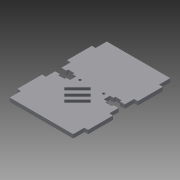
# Autodesk Inventor part: Motor_Mount_Front
Saved by Autodesk Inventor 2014 SP1 (Build 180222100, 222)
## iProperties
Created: 2014-03-20
Part Number: Motor_Mount_Front
Material: Generic
Document SubType Name: Modeling
Designer: ehagerup
Density: 1 g/cm^3
Appearance: Default
Author: ehagerup
Autodesk Inventor part; units mm, degrees
ref_plane "YZ Plane" through (0, 0, 0) normal (1, 0, 0) x (0, 1, 0)
ref_plane "XZ Plane" through (0, 0, 0) normal (0, 1, 0) x (-1, 0, 0)
ref_plane "XY Plane" through (0, 0, 0) normal (0, 0, 1) x (1, 0, 0)
sketch "Sketch1" plane through (0, 0, 0) normal (0, 0, 1) x (1, 0, 0)
  line L0 (0, 69) -> (3, 69)
  line L1 (3, 69) -> (3, 78)
  line L2 (3, 0) -> (3, 9)
  line L3 (3, 9) -> (0, 9)
  line L4 (0, 49) -> (3, 49)
  line L5 (3, 29) -> (0, 29)
  line L6 (15, 41.5) -> (15, 36.5)
  line L7 (12, 41.5) -> (12, 43)
  line L8 (12, 43) -> (7, 43)
  line L9 (7, 43) -> (7, 41.5)
  line L10 (12, 36.5) -> (12, 35)
  line L11 (12, 35) -> (7, 35)
  line L12 (7, 35) -> (7, 36.5)
  line L13 (0, 69) -> (0, 49)
  line L14 (0, 29) -> (0, 9)
  line L15 (3, 49) -> (3, 41.5)
  line L16 (3, 36.5) -> (3, 29)
  line L17 (15, 36.5) -> (12, 36.5)
  line L18 (7, 36.5) -> (3, 36.5)
  line L19 (3, 41.5) -> (7, 41.5)
  line L20 (12, 41.5) -> (15, 41.5)
  line L21 (57, 69) -> (54, 69)
  line L22 (54, 69) -> (54, 78)
  line L23 (54, 0) -> (54, 9)
  line L24 (54, 9) -> (57, 9)
  line L25 (57, 49) -> (54, 49)
  line L26 (54, 29) -> (57, 29)
  line L27 (42, 41.5) -> (42, 36.5)
  line L28 (45, 41.5) -> (45, 43)
  line L29 (45, 43) -> (50, 43)
  line L30 (50, 43) -> (50, 41.5)
  line L31 (45, 36.5) -> (45, 35)
  line L32 (45, 35) -> (50, 35)
  line L33 (50, 35) -> (50, 36.5)
  line L34 (57, 69) -> (57, 49)
  line L35 (57, 29) -> (57, 9)
  line L36 (54, 49) -> (54, 41.5)
  line L37 (54, 36.5) -> (54, 29)
  line L38 (42, 36.5) -> (45, 36.5)
  line L39 (50, 36.5) -> (54, 36.5)
  line L40 (54, 41.5) -> (50, 41.5)
  line L41 (45, 41.5) -> (42, 41.5)
  line L42 (3, 0) -> (54, 0)
  line L43 (54, 78) -> (3, 78)
  line L44 (24.2574, 22.636) -> (34.864, 33.2426)
  line L45 (34.864, 33.2426) -> (32.7426, 35.364)
  line L46 (32.7426, 35.364) -> (22.136, 24.7574)
  line L47 (22.136, 24.7574) -> (24.2574, 22.636)
  line L48 (20.0147, 26.8787) -> (30.6213, 37.4853)
  line L49 (30.6213, 37.4853) -> (28.5, 39.6066)
  line L50 (28.5, 39.6066) -> (17.8934, 29)
  line L51 (17.8934, 29) -> (20.0147, 26.8787)
  line L52 (28.5, 18.3934) -> (39.1066, 29)
  line L53 (39.1066, 29) -> (36.9853, 31.1213)
  line L54 (36.9853, 31.1213) -> (26.3787, 20.5147)
  line L55 (26.3787, 20.5147) -> (28.5, 18.3934)
  line L56 (24.2574, 22.636) -> (34.864, 33.2426)
  line L57 (34.864, 33.2426) -> (32.7426, 35.364)
  line L58 (32.7426, 35.364) -> (22.136, 24.7574)
  line L59 (22.136, 24.7574) -> (24.2574, 22.636)
  circle A0 centre (19, 40.5) radius 1
  circle A1 centre (38, 40.5) radius 1
  point P0 (0, 0)
  point P1 (57, 56.3821)
  point P2 (13.5, 36.5)
  point P3 (43.5, 41.5)
  dimension "d58" = 3
  dimension "d59" = 4
  dimension "d60" = 5
  dimension "d61" = 3
  dimension "d62" = 3
  dimension "d63" = 4
  dimension "d64" = 5
  dimension "d65" = 3
  dimension "d66" = 3
  dimension "d77" = 6
  dimension "d80" = 6
  dimension "d83" = 2
  dimension "d84" = 2
  dimension "d85" = 4
  dimension "d86" = 4
  dimension "d87" = 4
  dimension "d88" = 4
  constraints: 120 end point, 11 parallel, 6 horizontal, 6 perpendicular, 2 centre point, 2 collinear, 2 midpoint, 2 vertical, 1 point on line, 26 other
  measures "d58" distance between parallel lines of L7 L6
  measures "d59" distance between parallel lines of L15 L9
  measures "d60" distance of L7.end L8.end
  measures "d61" distance of L4.start L4.end
  measures "d62" distance of L5.start L5.end
  measures "d63" distance of L12.end L16.start
  measures "d64" distance of L10.end L11.end
  measures "d65" distance of L6.end L10.start
  measures "d66" distance of L0.start L0.end
  measures "d77" distance of L46.end L51.start
  measures "d80" distance of L46.end L55.start
  measures "d83" diameter of A1
  measures "d84" diameter of A0
  measures "d85" distance from line of L6 A0.centre
  measures "d86" distance from line of L27 A1.centre
  measures "d87" distance from line of L38 A1.centre
  measures "d88" distance from line of A0.centre L17
extrude "Extrusion1" add sketch "Sketch1" along normal blind 3
body "Solid1"
